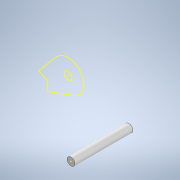
# Autodesk Inventor part: ReverserClicker
Saved by Autodesk Inventor 2021 (Build 250183000, 183)
## iProperties
Created: 2021-07-19
Part Number: ReverserClicker
Material: Generic
Document SubType Name: Modeling
Designer: teh18
Density: 1 g/cm^3
Appearance: Default
Author: teh18
Autodesk Inventor part; units mm, degrees
ref_plane "YZ Plane" through (0, 0, 0) normal (1, 0, 0) x (0, 1, 0)
ref_plane "XZ Plane" through (0, 0, 0) normal (0, 1, 0) x (-1, 0, 0)
ref_plane "XY Plane" through (0, 0, 0) normal (0, 0, 1) x (1, 0, 0)
sketch "Sketch1" plane through (0, 0, 0) normal (0, 0, 1) x (1, 0, 0)
  circle A0 centre (0, 0) radius 3.75
  dimension "d0" = 7.5
  constraints: 1 centre point, 1 coincident
  measures "d0" diameter of A0
ref_plane "Work Plane1" through (-31.2086, 47.0839, 55.625) normal (0, 0, 1) x (1, 0, 0)
ref_plane "Work Plane2" through (-28.2086, 47.0839, 35.0383) normal (0, 0, -1) x (0, 1, 0)
extrude "Extrusion1" add sketch "Sketch1" along normal up to surface (35.0383 mm away)
sketch "Sketch2" plane through (0, 0, 35.0383) normal (0, 0, 1) x (1, 0, 0)
  arc A0 (5.1057, 55.9273) -> (-11.4738, 79.6934) centre (0, 70.0316) ccw projected
  line L0 (-11.4738, 79.6934) -> (-28.2086, 59.8201) projected
  line L1 (-28.2086, 59.8201) -> (-20.0895, 56.0169) projected
  line L2 (-20.0895, 56.0169) -> (-19.3236, 47.0839) projected
  line L3 (-19.3236, 47.0839) -> (5.1057, 55.9273) projected
  circle A1 centre (0, 70.0316) radius 3.75 projected
  arc A2 (-75.9549, -10.8999) -> (-73.5792, -9.6288) centre (-75.4644, -8.9609) ccw projected
  arc A3 (-60.0244, -11.1884) -> (-73.5792, -9.6288) centre (-66.981, -11.9662) ccw projected
  arc A4 (-60.0244, -11.1884) -> (-56.998, -10.3955) centre (-67.3725, 23.0316) ccw projected
  line L4 (-56.998, -10.3955) -> (-59.9621, -0.8449) projected
  arc A5 (-59.9621, -0.8449) -> (-52.3252, 42.996) centre (-67.3725, 23.0316) ccw projected
  line L5 (-52.3252, 42.996) -> (-43.825, 48.9259) projected
  arc A6 (-43.825, 48.9259) -> (-87.3977, 51.7368) centre (-67.3725, 23.0316) ccw projected
  line L6 (-87.3977, 51.7368) -> (-93.1192, 59.9383) projected
  arc A7 (-93.1192, 59.9383) -> (-111.0378, 33.9101) centre (-67.3725, 23.0316) ccw projected
  line L7 (-111.0378, 33.9101) -> (-101.3344, 31.4926) projected
  arc A8 (-101.3344, 31.4926) -> (-101.7483, 29.6124) centre (-67.3725, 23.0316) ccw projected
  arc A9 (-99.8859, 16.0958) -> (-101.7483, 29.6124) centre (-102.3703, 22.6401) ccw projected
  arc A10 (-99.8859, 16.0958) -> (-101.1035, 13.6924) centre (-99.176, 14.226) ccw projected
  arc A11 (-101.1035, 13.6924) -> (-101.0492, 13.4984) centre (-67.3725, 23.0316) ccw projected
  arc A12 (-101.0492, 13.4984) -> (-98.7606, 12.0766) centre (-99.1248, 14.0431) ccw projected
  arc A13 (-92.062, 0.7684) -> (-98.7606, 12.0766) centre (-97.4858, 5.1936) ccw projected
  arc A14 (-92.062, 0.7684) -> (-91.9148, -1.9219) centre (-90.5124, -0.496) ccw projected
  arc A15 (-91.9148, -1.9219) -> (-91.7708, -2.0627) centre (-67.3725, 23.0316) ccw projected
  arc A16 (-91.7708, -2.0627) -> (-89.0779, -2.1498) centre (-90.3766, -0.6288) ccw projected
  arc A17 (-77.6226, -8.5937) -> (-89.0779, -2.1498) centre (-84.5324, -7.4732) ccw projected
  arc A18 (-77.6226, -8.5937) -> (-76.15, -10.8499) centre (-75.6484, -8.9138) ccw projected
  arc A19 (-76.15, -10.8499) -> (-75.9549, -10.8999) centre (-67.3725, 23.0316) ccw projected
  circle A20 centre (-67.3725, 23.0316) radius 18 projected
  line L8 (-47.5939, 41.5631) -> (-12.5105, -8.7275)
  circle A21 centre (0, 0) radius 15.2539
  line L9 (12.5105, 8.7275) -> (-27.0692, 45.961)
  line L10 (-19.6792, 51.2311) -> (-27.0692, 45.961)
  line L11 (-24.1491, 57.9185) -> (-47.5939, 41.5631)
  line L12 (-19.6792, 51.2311) -> (-20.0895, 56.0169)
  line L13 (-20.0895, 56.0169) -> (-24.1491, 57.9185)
  point P0 (0, 0)
  constraints: 12 end point, 2 collinear, 2 point on circle, 1 centre point, 1 coincident, 1 midpoint, 1 parallel, 1 perpendicular, 1 point on line, 1 tangent
extrude "Extrusion2" add sketch "Sketch2" along normal blind 10 contours L10 L9 A21 L8 L11 L1 L2 | L9 A21 picked at (4.0822, 2.4326)
body "Solid1"
